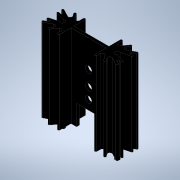
# Autodesk Inventor part: Steren Heatsink
Saved by Autodesk Inventor 2020.5 (Build 245400000, 400)
## iProperties
Created: 2022-12-14
Part Number: Steren Heatsink
Material: Aluminum 6061
Document SubType Name: Modeling
Designer: aivel
Density: 2.7 g/cm^3
Appearance: Anodized - Black
Author: aivel
Autodesk Inventor part; units mm, degrees
ref_plane "YZ Plane" through (0, 0, 0) normal (1, 0, 0) x (0, 1, 0)
ref_plane "XZ Plane" through (0, 0, 0) normal (0, 1, 0) x (-1, 0, 0)
ref_plane "XY Plane" through (0, 0, 0) normal (0, 0, 1) x (1, 0, 0)
sketch "Sketch1" plane through (0, 0, 0) normal (0, 1, 0) x (-1, 0, 0)
  line L0 (-9.35, 0) -> (-9.35, -12.5) construction
  line L1 (-25.4, 0) -> (-25.4, -12.5) construction
  line L2 (-9.35, -6.9) -> (-25.4, -6.9)
  line L3 (-25.4, -6.9) -> (-25.4, -5.6)
  line L4 (-25.4, -5.6) -> (-9.35, -5.6)
  line L5 (-9.35, -5.6) -> (-9.35, -6.9)
  circle A0 centre (-4.875, -6.25) radius 1
  circle A1 centre (-29.875, -6.25) radius 1
  line L6 (-9.35, 0) -> (-8.9, 0) construction
  line L7 (-25.4, 0) -> (-25.85, 0) construction
  line L8 (-8.45, -10.4049) -> (-8.45, -12.05)
  line L9 (-9.35, -12.05) -> (-9.35, -0.45)
  arc A2 (-8.45, -0.45) -> (-9.35, -0.45) centre (-8.9, -0.45) ccw
  arc A3 (-9.35, -12.05) -> (-8.45, -12.05) centre (-8.9, -12.05) ccw
  line L10 (-25.4, -12.05) -> (-25.4, -0.45)
  arc A4 (-25.4, -0.45) -> (-26.3, -0.45) centre (-25.85, -0.45) ccw
  arc A5 (-26.3, -12.05) -> (-25.4, -12.05) centre (-25.85, -12.05) ccw
  line L11 (-6.8219, -9.8759) -> (-4.9877, -12.4004)
  line L12 (-4.2596, -11.8714) -> (-5.0989, -10.7162)
  arc A6 (-4.9877, -12.4004) -> (-4.2596, -11.8714) centre (-4.6236, -12.1359) ccw
  line L13 (-3.9482, -9.3926) -> (-0.6086, -11.1683)
  line L14 (-0.1861, -10.3736) -> (-1.7142, -9.5611)
  arc A7 (-0.6086, -11.1683) -> (-0.1861, -10.3736) centre (-0.3973, -10.771) ccw
  line L15 (-1.3864, -8.7291) -> (-0.5511, -8.9529)
  line L16 (-0.3182, -8.0836) -> (-8.3489, -5.9318)
  arc A8 (-0.5511, -8.9529) -> (-0.3182, -8.0836) centre (-0.4347, -8.5183) ccw
  arc A9 (-6.8219, -9.8759) -> (-8.45, -10.4049) centre (-7.55, -10.4049) ccw
  arc A10 (-3.9482, -9.3926) -> (-5.0989, -10.7162) centre (-4.3708, -10.1872) ccw
  arc A11 (-1.3864, -8.7291) -> (-1.7142, -9.5611) centre (-1.5029, -9.1638) ccw
  line L17 (-8.45, -2.0951) -> (-8.45, -0.45)
  line L18 (-6.8219, -2.6241) -> (-4.9877, -0.0996)
  line L19 (-4.2596, -0.6286) -> (-5.0989, -1.7838)
  arc A12 (-4.2596, -0.6286) -> (-4.9877, -0.0996) centre (-4.6236, -0.3641) ccw
  line L20 (-3.9482, -3.1074) -> (-0.6086, -1.3317)
  line L21 (-0.1861, -2.1264) -> (-1.7142, -2.9389)
  arc A13 (-0.1861, -2.1264) -> (-0.6086, -1.3317) centre (-0.3973, -1.729) ccw
  line L22 (-1.3864, -3.7709) -> (-0.5511, -3.5471)
  line L23 (-0.3182, -4.4164) -> (-8.3489, -6.5682)
  arc A14 (-0.3182, -4.4164) -> (-0.5511, -3.5471) centre (-0.4347, -3.9817) ccw
  arc A15 (-8.45, -2.0951) -> (-6.8219, -2.6241) centre (-7.55, -2.0951) ccw
  arc A16 (-5.0989, -1.7838) -> (-3.9482, -3.1074) centre (-4.3708, -2.3128) ccw
  arc A17 (-1.7142, -2.9389) -> (-1.3864, -3.7709) centre (-1.5029, -3.3362) ccw
  line L24 (-26.3, -10.4049) -> (-26.3, -12.05)
  arc A18 (-26.3, -12.05) -> (-25.4, -12.05) centre (-25.85, -12.05) ccw
  line L25 (-27.9281, -9.8759) -> (-29.7623, -12.4004)
  line L26 (-30.4904, -11.8714) -> (-29.6511, -10.7162)
  arc A19 (-30.4904, -11.8714) -> (-29.7623, -12.4004) centre (-30.1264, -12.1359) ccw
  line L27 (-30.8018, -9.3926) -> (-34.1414, -11.1683)
  line L28 (-34.5639, -10.3736) -> (-33.0358, -9.5611)
  arc A20 (-34.5639, -10.3736) -> (-34.1414, -11.1683) centre (-34.3527, -10.771) ccw
  line L29 (-33.3636, -8.7291) -> (-34.1989, -8.9529)
  line L30 (-34.4318, -8.0836) -> (-26.4011, -5.9318)
  arc A21 (-34.4318, -8.0836) -> (-34.1989, -8.9529) centre (-34.3153, -8.5183) ccw
  arc A22 (-26.3, -10.4049) -> (-27.9281, -9.8759) centre (-27.2, -10.4049) ccw
  arc A23 (-29.6511, -10.7162) -> (-30.8018, -9.3926) centre (-30.3792, -10.1872) ccw
  arc A24 (-33.0358, -9.5611) -> (-33.3636, -8.7291) centre (-33.2471, -9.1638) ccw
  line L31 (-26.3, -2.0951) -> (-26.3, -0.45)
  arc A25 (-27.9281, -2.6241) -> (-26.3, -2.0951) centre (-27.2, -2.0951) ccw
  line L32 (-27.9281, -2.6241) -> (-29.7623, -0.0996)
  arc A26 (-29.7623, -0.0996) -> (-30.4904, -0.6286) centre (-30.1264, -0.3641) ccw
  line L33 (-30.4904, -0.6286) -> (-29.6511, -1.7838)
  arc A27 (-30.8018, -3.1074) -> (-29.6511, -1.7838) centre (-30.3792, -2.3128) ccw
  line L34 (-30.8018, -3.1074) -> (-34.1414, -1.3317)
  arc A28 (-34.1414, -1.3317) -> (-34.5639, -2.1264) centre (-34.3527, -1.729) ccw
  line L35 (-34.5639, -2.1264) -> (-33.0358, -2.9389)
  arc A29 (-33.3636, -3.7709) -> (-33.0358, -2.9389) centre (-33.2471, -3.3362) ccw
  line L36 (-33.3636, -3.7709) -> (-34.1989, -3.5471)
  arc A30 (-34.1989, -3.5471) -> (-34.4318, -4.4164) centre (-34.3153, -3.9817) ccw
  line L37 (-34.4318, -4.4164) -> (-26.4011, -6.5682)
  point P0 (0, 0)
  point P1 (-25.85, -6.25)
  point P2 (-6.6296, -9.375)
  point P3 (-4.45, -8.6161)
  point P4 (-4.45, -7.4424)
  point P5 (-30.5005, -5.4698)
  point P6 (-30.5005, -7.0302)
  point P7 (-4.2495, -7.0302)
  point P8 (-4.2495, -5.4698)
  constraints: 76 end point, 60 point on circle, 31 centre point, 18 tangent, 6 parallel, 3 point on line, 1 horizontal, 1 perpendicular
extrude "Extrusion1" add sketch "Sketch1" along normal blind 38 contours L2 L3 L4 L5 | L5 L9 A2 L17 A15 L18 A12 L19 A16 L20 A13 L21 A17 L22 A14 L23 A0 L16 A8 L15 A11 L14 A7 L13 A10 L12 A6 L11 A9 L8 A3 | L10 A5 L24 A22 L25 A19 L26 A23 L27 A20 L28 A24 L29 A21 L30 A1 L37 A30 L36 A29 L35 A28 L34 A27 L33 A26 L32 A25 L31 A4 L3 | L16 L23 A0 | A1 L37 L30 picked at (-6.2987, -6.25) picked at (-28.4488, -6.2912)
extrude "Extrusion2" add sketch "Sketch1" along normal blind 8 and the other way blind 4 contours L16 A0 L23 | A0 L16 | L30 A1 | A1 L37 L30 | L23 A0 | A1 L37 picked at (-4.6521, -6.705) picked at (-30.1259, -6.0659)
sketch "Sketch2" plane through (9.35, 0, -5.6) normal (0, 0, 1) x (1, 0, 0)
  line L0 (0, 0) -> (16.05, 0) construction
  line L1 (8.025, 0) -> (13.525, 0) construction
  line L2 (13.525, 0) -> (2.525, 0)
  line L3 (2.525, 0) -> (2.525, 9.3)
  line L4 (2.525, 9.3) -> (13.525, 9.3)
  line L5 (13.525, 9.3) -> (13.525, 0)
  line L6 (0, 38) -> (16.05, 38) construction
  circle A0 centre (8.025, 25.5) radius 1.5
  circle A1 centre (8.025, 18.5) radius 1.5
  circle A2 centre (8.025, 13.5) radius 1.5
  point P0 (-9.35, 0)
  constraints: 10 end point, 3 centre point, 2 parallel, 1 horizontal, 1 midpoint, 1 perpendicular, 1 point on line
extrude "Extrusion3" cut sketch "Sketch2" against normal through all
body "Solid1"
